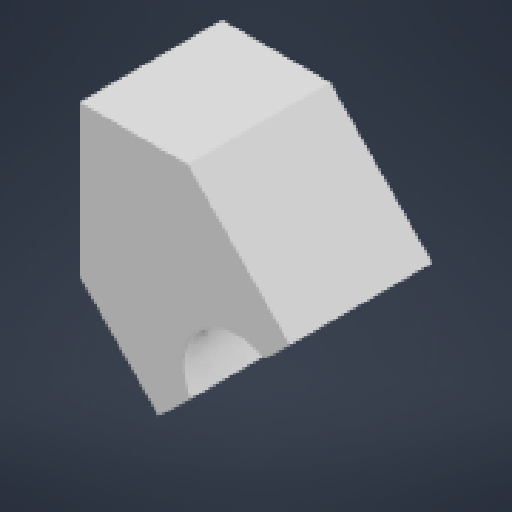
# Autodesk Inventor part: back cpap holder and pg
Saved by Autodesk Inventor 2024.3 (Build 283343000, 343)
## iProperties
Created: 2024-11-28
Part Number: back cpap holder and pg
Material: Generic
Document SubType Name: Modeling
Designer: MFil
Density: 1 g/cm^3
Appearance: Default
Author: MFil
Autodesk Inventor part; units mm, degrees
ref_plane "YZ Plane" through (0, 0, 0) normal (1, 0, 0) x (0, 1, 0)
ref_plane "XZ Plane" through (0, 0, 0) normal (0, 1, 0) x (-1, 0, 0)
ref_plane "XY Plane" through (0, 0, 0) normal (0, 0, 1) x (1, 0, 0)
sketch "Sketch1" plane through (0, 0, 0) normal (0, 0, 1) x (1, 0, 0)
  circle A0 centre (-22.95, -2.7) radius 1.7 projected
  circle A1 centre (-6.95, -2.7) radius 1.7 projected
  circle A2 centre (-22.95, -2.7) radius 4.7
  circle A3 centre (-6.95, -2.7) radius 3.7
  line L0 (3.4322, -7.8015) -> (-0.1118, -11.233) projected
  line L1 (6.9476, -1.614) -> (-26.719, -34.211)
  line L2 (-14.4322, -25.0985) -> (-13.041, -26.5353) projected
  line L3 (-12.4947, -28.5372) -> (-38.4967, -1.682)
  line L4 (-27.65, -2.7) -> (-27.65, -12.8846)
  arc A4 (-10.8882, -21.667) -> (-0.1118, -11.233) centre (-5.5, -16.45) ccw projected
  line L5 (-5.5, -16.45) -> (-6.8912, -15.0131)
  line L6 (-27.65, -2.7) -> (-22.95, -2.7)
  line L7 (-2.8497, 4.7907) -> (-5.9286, 4.7907) construction
  line L8 (1, 3.7907) -> (-32.1675, 3.7907)
  line L9 (1.89, -6.5109) -> (-12.4504, 8.3)
  line L10 (-12.4504, 8.3) -> (-43.44, 8.3)
  line L11 (-27.65, 8.3) -> (-27.65, -2.7)
  circle A5 centre (-5.5, -16.45) radius 7.5
  point P0 (0, 0)
  point P1 (-22.95, 2)
  point P2 (-6.95, 1)
  point P3 (-3.8133, -0.7376)
  point P4 (2.6084, -5.8153)
  point P5 (-13.7366, -25.8169)
  point P6 (-16.5419, -24.3572)
  point P7 (-4.3892, 4.7907)
  point P8 (-6.8365, 3.7907)
  point P9 (-27.65, 3.7907)
  point P10 (-4.2918, -0.1263)
  point P11 (-12.0843, -20.0413)
  point P12 (-1.6981, -9.985)
  dimension "d0" = 3
  dimension "d1" = 2
  dimension "d2" = 2
  dimension "d3" = 1
  dimension "d9" = 1
  dimension "d10" = 11
  constraints: 18 end point, 7 point on line, 4 point on circle, 3 centre point, 3 tangent, 2 horizontal, 2 midpoint, 2 parallel, 2 perpendicular, 1 coincident, 1 collinear, 1 vertical
  measures "d0" radial gap between concentric circles of A0 A2
  measures "d1" radial gap between concentric circles of A1 A3
  measures "d2" distance between parallel lines of L0 L1
  measures "d3" distance from line of point (-13.737, -25.817) L3
  measures "d9" distance from line of L8 point (-4.389, 4.791)
  measures "d10" distance from line of A0.centre L10
extrude "Extrusion1" add sketch "Sketch1" along normal blind 20 contours A0 | A2 | A3 | L11 L8 L9 L1 A5 L3 L4 | L11 L10 L9 L8 | A1
body "Solid1"
